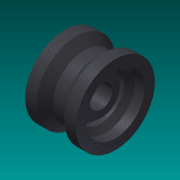
# Autodesk Inventor part: pulley
Saved by Autodesk Inventor 2014 SP2 (Build 180246200, 246)
## iProperties
Created: 2019-06-27
Part Number: pulley
Material: Iron, Cast
Document SubType Name: Modeling
Designer: USER PC
Density: 7.25 g/cm^3
Appearance: Iron - Cast
Author: USER PC
Autodesk Inventor part; units mm, degrees
ref_plane "YZ Plane" through (0, 0, 0) normal (1, 0, 0) x (0, 1, 0)
ref_plane "XZ Plane" through (0, 0, 0) normal (0, 1, 0) x (-1, 0, 0)
ref_plane "XY Plane" through (0, 0, 0) normal (0, 0, 1) x (1, 0, 0)
sketch "Sketch1" plane through (0, 0, 0) normal (0, 0, 1) x (1, 0, 0)
  line L0 (0, 0) -> (0, 20)
  line L1 (0, 20) -> (0, 70) construction
  line L2 (0, 20) -> (20, 20)
  line L3 (20, 20) -> (20, 33)
  line L4 (20, 33) -> (8, 33)
  line L5 (8, 33) -> (8, 43)
  line L6 (45, 52.057) -> (45, 70)
  line L7 (10, 56.0449) -> (0, 56.0449)
  line L8 (-63, 0) -> (63, 0) projected
  line L9 (45, 70) -> (25, 70)
  line L10 (45, 52.057) -> (27.7352, 52.057)
  line L11 (8, 43) -> (18, 43)
  line L12 (18, 43) -> (27.7352, 52.057)
  line L13 (10, 56.0449) -> (25, 70)
  line L14 (0, 20) -> (-20, 20)
  line L15 (-20, 20) -> (-20, 33)
  line L16 (-20, 33) -> (-8, 33)
  line L17 (-8, 33) -> (-8, 43)
  line L18 (-45, 52.057) -> (-45, 70)
  line L19 (-10, 56.0449) -> (0, 56.0449)
  line L20 (-45, 70) -> (-25, 70)
  line L21 (-45, 52.057) -> (-27.7352, 52.057)
  line L22 (-8, 43) -> (-18, 43)
  line L23 (-18, 43) -> (-27.7352, 52.057)
  line L24 (-10, 56.0449) -> (-25, 70)
  dimension "d3" = 20
  dimension "d5" = 10
  dimension "d9" = 45
  dimension "d11" = 8
  dimension "d12" = 20
  dimension "d13" = 10
  dimension "d14" = 15
  dimension "d16" = 20
  dimension "d17" = 70
  dimension "d18" = 10
  dimension "d19" = 13
  constraints: 48 end point, 10 symmetric about line, 5 perpendicular, 4 parallel, 1 collinear, 1 point on line, 1 vertical
  measures "d3" distance of L0.end L2.end
  measures "d5" distance of L7.start L7.end
  measures "d9" distance between parallel lines of L6 L1
  measures "d11" distance between parallel lines of L5 L1
  measures "d12" distance of L6.end L9.end
  measures "d13" distance of L5.end L11.end
  measures "d14" distance between parallel lines of L12 L13
  measures "d16" horizontal distance of L0.start L2.end
  measures "d17" vertical distance of L0.start L6.end
  measures "d18" distance of L4.end L5.end
  measures "d19" distance of L2.end L3.end
revolve "Revolution2" add sketch "Sketch1" angle 360 about axis through (-10, 0, 0) along (1, 0, 0)
body "Solid2"
